Autodesk Fusion 360 part; units mm, degrees
(part 2 of 2)
extrude "Extrude1" add sketch "Sketch1" against normal blind 0.5 contours L0 L1 L2 L3 L4 L5 L6 L7 L8 L315 L316 | L18 L19 L20 L21 L38 L39 L40 L41 L42 L43 L44 L45 L46 L47 L48 L49 L50 L51 L52 L53 L54 L55 L56 L57 L58 L59 L60 L61 L62 L63 L64 L65 L66 L67 L68 L69 L70 L71 L72 L73 L74 L75 L76 L77 L78 L79 L80 L81 L82 L83 L84 L85 L86 L87 L88 L89 L90 L190 L191 L192 L193 L194 L195 L196 L197 L198 L199 L200 L201 L202 L203 L204 L205 L206 L207 L208 L209 L210 L211 L271 L272 L273 L274 L275 L276 L277 L278 L279 L280 L281 L282 L295 L296 L297 L298 L299 L300 L301 L313 L314 L315 L316 L329 L330 L331 L332 L333 L334 L335 L336 L337 L338 L339 L340 L341 L342 L343 L344 L345 L346 L347 L348 L349 L350 L351 L352 L353 L354 L355 L356 L357 L358 L359 L360 L361 L362 L363 L364 L411 L412 L413 L414 L415 L416 L417 L418 L419 L420 L421 L422 L423 L424 L425 L426 L427 L428 L429 L430 L431 L473 L474 L475 L476 L477 L478 L479 L480 L481 L482 L483 L484 L485 L486 L487 L488 L489 L490 L491 L492 L493 L494 L495 L496 L497 L498 L499 L500 L572 L573 L574 L575 L576 L577 L578 L579 L580 L581 L582 L583 L596 L597 L598 L599 L600 L601 L602 L603 L604 L605 L606 L607 L608 L609 L610 L611 L612 L613 L614 L615 L616 L617 L619 | L10 L11 L12 L316 | L313 L316 L317 L318 L319 L320 L321 L322 L323 L324 L325 L326 | L314 L620 L621 L622 L623 L624 L625 L626 L627 L628 L629 L630 L631 L632 | L313 L453 L454 L455 | L313 L314 L634 L635 L636 L637 L638 L639 | L313 L557 L558 L559 L560 L561 L562 L563 L564 L565 L566 L567 L568 L569 L570 L571 | L169 L170 L171 L172 L173 L174 L175 L176 L177 L178 L179 L180 L181 L182 L183 L184 L185 L186 L187 L188 L189 | L246 L247 L248 L249 L250 L251 L252 L253 | L263 L264 L265 L266 L267 L268 L269 L270 | L461 L462 L463 L464 L465 L466 L467 L468 L469 L470 L471 L472 | L692 L693 L694 L695 L696 L697 L702 L703 | L698 L699 L700 L701 makes body 1 at (43.6667, 42, 0) makes body 2 at (43.6667, 30.6667, 0) makes body 3 at (24, 8.3333, 0) makes body 4 at (55.6667, 34.6667, 0) makes body 5 at (24.3333, 29, 0)
extrude "Extrude2" add sketch "Sketch1" along normal blind 1 separate body contours L1 L2 L3 L4 L5 L6 L7 L8 L9 L10 L11 L12 L13 L14 L18 L19 L20 L21 L315 L316 | L38 L39 L40 L41 L42 L43 L44 L45 L46 L47 L48 L49 L50 L51 L52 L53 L54 L55 L56 L57 L58 L59 L60 L61 L62 L63 L64 L65 L66 L67 L68 L69 L70 L71 L72 L73 L74 L75 L76 L77 L78 L79 L80 L81 L82 L83 L84 L85 L86 L87 L88 L89 L90 L315 | L191 L192 L193 L194 L195 L196 L197 L198 L199 L200 L201 L202 L203 L204 L205 L206 L207 L208 L209 L210 L211 L315 | L313 L316 L319 L320 L321 L322 L323 L324 L325 L326 L327 L328 L329 L330 L331 L332 L333 L334 L335 L336 L337 L338 L339 L340 L341 L342 L343 L344 L345 L346 L347 L348 L349 L350 L351 L352 L353 L354 L355 L356 L357 L358 L359 L360 L361 L362 L363 L364 | L272 L273 L274 L275 L276 L277 L278 L279 L280 L281 L282 L315 | L295 L296 L297 L298 L299 L300 L301 L302 L303 L314 L315 | L313 L314 L597 L598 L599 L600 L601 L602 L603 L604 L605 L606 L607 L608 L609 L610 L611 L612 L613 L614 L615 L616 L617 L618 L619 L620 L621 L622 L623 L624 L625 L626 L627 L628 L629 L630 L631 L632 L633 L634 L635 L636 L637 L638 L639 | L313 L413 L414 L415 L416 L417 L418 L419 L420 L421 L422 L423 L424 L425 L426 L427 L428 L429 L430 L431 L453 L454 L455 | L313 L474 L475 L476 L477 L478 L479 L480 L481 L482 L483 L484 L485 L486 L487 L488 L489 L490 L491 L492 L493 L494 L495 L496 L497 L498 L499 L500 L557 L558 L559 L560 L561 L562 L563 L564 L565 L566 L567 L568 L569 L570 L571 | L313 L573 L574 L575 L576 L577 L578 L579 L580 L581 L582 L583 | L147 L148 L149 L150 L151 L152 L153 L154 L155 L156 L157 L158 L159 L160 L161 L162 L163 L164 L165 L166 L167 L168 | L238 L239 L240 L241 L242 L243 L244 L245 | L254 L255 L256 L257 L258 L259 L260 L261 L262 makes body 6 at (32.3333, 5, 0) makes body 7 at (63.3333, 32.3333, 0) makes body 8 at (21.3333, 30, 0) makes body 9 at (22, 36, 0) makes body 10 at (39.3333, 31, 0) makes body 11 at (54.3333, 6.3333, 0) makes body 12 at (18.3333, 5, 0) makes body 13 at (74.3333, 29.3333, 0) makes body 14 at (42.3333, 31, 0) makes body 15 at (1, 43, 0) makes body 16 at (42.3333, 40.6667, 0) makes body 17 at (76, 0.3333, 0) makes body 18 at (0.3333, 7.6667, 0)
extrude "Extrude3" cut sketch "Sketch1" against normal blind 1 contours L461 L462 L463 L464 L465 L466 L467 L468 L469 L470 L471 L472 bodies 3
extrude "Extrude4" add sketch "Sketch1" along normal blind 1 separate body contours L461 L462 L463 L464 L465 L466 L467 L468 L469 L470 L471 L472 makes body 19
extrude "Extrude5" add sketch "Sketch1" against normal blind 1 separate body contours L15 L16 L17 L22 L23 L24 L25 L26 L27 L28 L29 L30 L31 L32 L33 L34 L35 L36 L37 | L91 L92 L93 L94 L95 L96 L97 L98 L99 L100 L101 L102 L103 L104 L105 L106 L107 L108 L109 L110 L111 L112 L113 L114 L115 L116 L117 L118 L119 L120 L121 L122 L123 L124 L125 L126 L127 L128 L129 L130 L131 L132 L133 L134 L135 L136 L137 L138 L139 L140 L141 L142 L143 L144 L145 L146 | L212 L213 L214 L215 L216 L217 L218 L219 L220 L221 L222 L223 L224 L225 L226 L227 L228 L229 L230 L231 L232 L233 L234 L235 L236 L237 | L283 L284 L285 L286 L287 L288 L289 L290 L291 L292 L293 L294 | L304 L305 L306 L307 L308 L309 L310 L311 L312 | L365 L366 L367 L368 L369 L370 L371 L372 L373 L374 L375 L376 L377 L378 L379 L380 L381 L382 L383 L384 L385 L386 L387 L388 L389 L390 L391 L392 L393 L394 L395 L396 L397 L398 L399 L400 L401 L402 L403 L404 L405 L406 L407 L408 L409 L410 | L432 L433 L434 L435 L436 L437 L438 L439 L440 L441 L442 L443 L444 L445 L446 L447 L448 L449 L450 L451 L452 L456 L457 L458 L459 L460 | L501 L502 L503 L504 L505 L506 L507 L508 L509 L510 L511 L512 L513 L514 L515 L516 L517 L518 L519 L520 L521 L522 L523 L524 L525 L526 L527 L528 L529 L530 L531 L532 L533 L534 L535 L536 L537 L538 L539 L540 L541 L542 L543 L544 L545 L546 L547 L548 L549 L550 L551 L552 L553 L554 L555 L556 | L584 L585 L586 L587 L588 L589 L590 L591 L592 L593 L594 L595 | L640 L641 L642 L643 L644 L645 L646 L647 L648 L649 L650 L651 L652 L653 L654 L655 L656 L657 L658 L659 L660 L661 L662 L663 L664 L665 L666 L667 L668 L669 L670 L671 L672 L673 L674 L675 L676 L677 L678 L679 L680 L681 L682 L683 L684 L685 L686 L687 L688 L689 L690 L691 makes body 20 at (76, 46, 0) makes body 21 at (19, 35.3333, 0) makes body 22 at (19.6667, 6.6667, 0) makes body 23 at (9, 38.6667, 0) makes body 24 at (55.6667, 8.6667, 0) makes body 25 at (60.3333, 38, 0) makes body 26 at (34, 5, 0) makes body 27 at (11, 9.3333, 0) makes body 28 at (43, 24, 0) makes body 29 at (73, 2, 0)
extrude "Extrude6" add 14 faces at (1, 43, 0) (22, 36, 0) (21.3333, 30, 0) (39.3333, 31, 0) (42.3333, 31, 0) (42.3333, 40.6667, 0) (63.3333, 32.3333, 0) (74.3333, 29.3333, 0) (76, 0.3333, 0) (54.3333, 6.3333, 0) (32.3333, 5, 0) (21.3333, 10.3333, 0) (18.3333, 5, 0) (0.3333, 7.6667, 0) along direction (0, 0, -1) blind 0.5 on bodies 6 7 8 9 10 11 12 13 14 15 16 17 18 19 bodies 15 1 2 3 4 5 6 7 8 9 10 11 12 13 14 16 17 18 19 20 21 22 23 24 25 26 27 28 29
extrude "Extrude7" cut 10 faces at (11, 9.3333, -1) (19.6667, 6.6667, -1) (34, 5, -1) (55.6667, 8.6667, -1) (73, 2, -1) (60.3333, 38, -1) (76, 46, -1) (43, 24, -1) (19, 35.3333, -1) (9, 38.6667, -1) along direction (0, 0, 1) blind 0.5 on bodies 15 bodies 15
sketch "Sketch2" plane through (0, 0, 0) normal (0, 0, 1) x (1, 0, 0)
  line L0 (1, 14) -> (1, 15)
  line L1 (1, 15) -> (2, 15)
  line L2 (2, 15) -> (2, 16)
  line L3 (2, 16) -> (3, 16)
  line L4 (3, 16) -> (3, 17)
  line L5 (3, 17) -> (4, 17)
  line L6 (4, 17) -> (4, 18)
  line L7 (4, 18) -> (11, 18)
  line L8 (11, 18) -> (11, 14)
  line L9 (11, 14) -> (6, 14)
  line L10 (6, 14) -> (6, 13)
  line L11 (6, 13) -> (5, 13)
  line L12 (5, 13) -> (5, 12)
  line L13 (5, 12) -> (4, 12)
  line L14 (4, 12) -> (4, 6)
  line L15 (4, 6) -> (5, 6)
  line L16 (5, 6) -> (5, 5)
  line L17 (5, 5) -> (6, 5)
  line L18 (6, 5) -> (6, 4)
  line L19 (6, 4) -> (9, 4)
  line L20 (9, 4) -> (9, 5)
  line L21 (9, 5) -> (10, 5)
  line L22 (10, 5) -> (10, 6)
  line L23 (10, 6) -> (11, 6)
  line L24 (11, 6) -> (11, 7)
  line L25 (11, 7) -> (7, 7)
  line L26 (7, 7) -> (7, 11)
  line L27 (7, 11) -> (14, 11)
  line L28 (14, 11) -> (14, 3)
  line L29 (14, 3) -> (13, 3)
  line L30 (13, 3) -> (13, 2)
  line L31 (13, 2) -> (12, 2)
  line L32 (12, 2) -> (12, 1)
  line L33 (12, 1) -> (11, 1)
  line L34 (11, 1) -> (11, 0)
  line L35 (11, 0) -> (4, 0)
  line L36 (4, 0) -> (4, 1)
  line L37 (4, 1) -> (3, 1)
  line L38 (3, 1) -> (3, 2)
  line L39 (3, 2) -> (2, 2)
  line L40 (2, 2) -> (2, 3)
  line L41 (2, 3) -> (1, 3)
  line L42 (1, 3) -> (1, 4)
  line L43 (1, 4) -> (0, 4)
  line L44 (0, 4) -> (0, 14)
  line L45 (0, 14) -> (1, 14)
  line L46 (54, 0) -> (54, 18)
  line L47 (54, 18) -> (65, 18)
  line L48 (65, 18) -> (65, 14)
  line L49 (65, 14) -> (58, 14)
  line L50 (58, 14) -> (58, 11)
  line L51 (58, 11) -> (61, 11)
  line L52 (61, 11) -> (61, 7)
  line L53 (61, 7) -> (58, 7)
  line L54 (58, 7) -> (58, 4)
  line L55 (58, 4) -> (65, 4)
  line L56 (65, 4) -> (65, 0)
  line L57 (65, 0) -> (54, 0)
  line L58 (70, 43) -> (70, 48)
  line L59 (70, 48) -> (83, 48)
  line L60 (83, 48) -> (83, 43)
  line L61 (83, 43) -> (79, 43)
  line L62 (79, 43) -> (79, 22)
  line L63 (79, 22) -> (74, 22)
  line L64 (74, 22) -> (74, 43)
  line L65 (74, 43) -> (70, 43)
  line L66 (17, 45) -> (18, 45)
  line L67 (18, 45) -> (18, 46)
  line L68 (18, 46) -> (19, 46)
  line L69 (19, 46) -> (19, 47)
  line L70 (19, 47) -> (20, 47)
  line L71 (20, 47) -> (20, 48)
  line L72 (20, 48) -> (30, 48)
  line L73 (30, 48) -> (30, 47)
  line L74 (30, 47) -> (31, 47)
  line L75 (31, 47) -> (31, 46)
  line L76 (31, 46) -> (32, 46)
  line L77 (32, 46) -> (32, 45)
  line L78 (32, 45) -> (33, 45)
  line L79 (33, 45) -> (33, 40)
  line L80 (33, 40) -> (28, 40)
  line L81 (28, 40) -> (28, 42)
  line L82 (28, 42) -> (27, 42)
  line L83 (27, 42) -> (27, 43)
  line L84 (27, 43) -> (24, 43)
  line L85 (24, 43) -> (24, 42)
  line L86 (24, 42) -> (23, 42)
  line L87 (23, 42) -> (23, 41)
  line L88 (23, 41) -> (22, 41)
  line L89 (22, 41) -> (22, 37)
  line L90 (22, 37) -> (23, 37)
  line L91 (23, 37) -> (23, 38)
  line L92 (23, 38) -> (29, 38)
  line L93 (29, 38) -> (29, 37)
  line L94 (29, 37) -> (30, 37)
  line L95 (30, 37) -> (30, 36)
  line L96 (30, 36) -> (31, 36)
  line L97 (31, 36) -> (31, 35)
  line L98 (31, 35) -> (32, 35)
  line L99 (32, 35) -> (32, 34)
  line L100 (32, 34) -> (33, 34)
  line L101 (33, 34) -> (33, 25)
  line L102 (33, 25) -> (32, 25)
  line L103 (32, 25) -> (32, 24)
  line L104 (32, 24) -> (31, 24)
  line L105 (31, 24) -> (31, 23)
  line L106 (31, 23) -> (30, 23)
  line L107 (30, 23) -> (30, 22)
  line L108 (30, 22) -> (21, 22)
  line L109 (21, 22) -> (21, 23)
  line L110 (21, 23) -> (20, 23)
  line L111 (20, 23) -> (20, 24)
  line L112 (20, 24) -> (19, 24)
  line L113 (19, 24) -> (19, 25)
  line L114 (19, 25) -> (18, 25)
  line L115 (18, 25) -> (18, 26)
  line L116 (18, 26) -> (17, 26)
  line L117 (17, 26) -> (17, 45)
  line L118 (54, 22) -> (54, 27)
  line L119 (54, 27) -> (58, 27)
  line L120 (58, 27) -> (58, 43)
  line L121 (58, 43) -> (54, 43)
  line L122 (54, 43) -> (54, 48)
  line L123 (54, 48) -> (68, 48)
  line L124 (68, 48) -> (68, 43)
  line L125 (68, 43) -> (64, 43)
  line L126 (64, 43) -> (64, 27)
  line L127 (64, 27) -> (68, 27)
  line L128 (68, 27) -> (68, 22)
  line L129 (68, 22) -> (54, 22)
  line L130 (83, 18) -> (83, 14)
  line L131 (83, 14) -> (74, 14)
  line L132 (74, 14) -> (74, 12)
  line L133 (74, 12) -> (75, 12)
  line L134 (75, 12) -> (75, 11)
  line L135 (75, 11) -> (79, 11)
  line L136 (79, 11) -> (79, 10)
  line L137 (79, 10) -> (80, 10)
  line L138 (80, 10) -> (80, 9)
  line L139 (80, 9) -> (81, 9)
  line L140 (81, 9) -> (81, 8)
  line L141 (81, 8) -> (82, 8)
  line L142 (82, 8) -> (82, 7)
  line L143 (82, 7) -> (83, 7)
  line L144 (83, 7) -> (83, 3)
  line L145 (83, 3) -> (82, 3)
  line L146 (82, 3) -> (82, 2)
  line L147 (82, 2) -> (81, 2)
  line L148 (81, 2) -> (81, 1)
  line L149 (81, 1) -> (80, 1)
  line L150 (80, 1) -> (80, 0)
  line L151 (80, 0) -> (69, 0)
  line L152 (69, 0) -> (69, 4)
  line L153 (69, 4) -> (78, 4)
  line L154 (78, 4) -> (78, 6)
  line L155 (78, 6) -> (77, 6)
  line L156 (77, 6) -> (77, 7)
  line L157 (77, 7) -> (73, 7)
  line L158 (73, 7) -> (73, 8)
  line L159 (73, 8) -> (72, 8)
  line L160 (72, 8) -> (72, 9)
  line L161 (72, 9) -> (71, 9)
  line L162 (71, 9) -> (71, 10)
  line L163 (71, 10) -> (70, 10)
  line L164 (70, 10) -> (70, 11)
  line L165 (70, 11) -> (69, 11)
  line L166 (69, 11) -> (69, 15)
  line L167 (69, 15) -> (70, 15)
  line L168 (70, 15) -> (70, 16)
  line L169 (70, 16) -> (71, 16)
  line L170 (71, 16) -> (71, 17)
  line L171 (71, 17) -> (72, 17)
  line L172 (72, 17) -> (72, 18)
  line L173 (72, 18) -> (83, 18)
  line L174 (47, 0) -> (47, 12)
  line L175 (47, 12) -> (46, 12)
  line L176 (46, 12) -> (46, 13)
  line L177 (46, 13) -> (44, 13)
  line L178 (44, 13) -> (44, 12)
  line L179 (44, 12) -> (43, 12)
  line L180 (43, 12) -> (43, 7)
  line L181 (43, 7) -> (40, 7)
  line L182 (40, 7) -> (40, 12)
  line L183 (40, 12) -> (39, 12)
  line L184 (39, 12) -> (39, 13)
  line L185 (39, 13) -> (37, 13)
  line L186 (37, 13) -> (37, 12)
  line L187 (37, 12) -> (36, 12)
  line L188 (36, 12) -> (36, 0)
  line L189 (36, 0) -> (32, 0)
  line L190 (32, 0) -> (32, 14)
  line L191 (32, 14) -> (33, 14)
  line L192 (33, 14) -> (33, 15)
  line L193 (33, 15) -> (34, 15)
  line L194 (34, 15) -> (34, 16)
  line L195 (34, 16) -> (35, 16)
  line L196 (35, 16) -> (35, 17)
  line L197 (35, 17) -> (36, 17)
  line L198 (36, 17) -> (36, 18)
  line L199 (36, 18) -> (40, 18)
  line L200 (40, 18) -> (40, 17)
  line L201 (40, 17) -> (41, 17)
  line L202 (41, 17) -> (41, 16)
  line L203 (41, 16) -> (42, 16)
  line L204 (42, 16) -> (42, 17)
  line L205 (42, 17) -> (43, 17)
  line L206 (43, 17) -> (43, 18)
  line L207 (43, 18) -> (47, 18)
  line L208 (47, 18) -> (47, 17)
  line L209 (47, 17) -> (48, 17)
  line L210 (48, 17) -> (48, 16)
  line L211 (48, 16) -> (49, 16)
  line L212 (49, 16) -> (49, 15)
  line L213 (49, 15) -> (50, 15)
  line L214 (50, 15) -> (50, 14)
  line L215 (50, 14) -> (51, 14)
  line L216 (51, 14) -> (51, 0)
  line L217 (51, 0) -> (47, 0)
  line L218 (18, 0) -> (18, 14)
  line L219 (18, 14) -> (19, 14)
  line L220 (19, 14) -> (19, 15)
  line L221 (19, 15) -> (20, 15)
  line L222 (20, 15) -> (20, 16)
  line L223 (20, 16) -> (21, 16)
  line L224 (21, 16) -> (21, 17)
  line L225 (21, 17) -> (22, 17)
  line L226 (22, 17) -> (22, 18)
  line L227 (22, 18) -> (25, 18)
  line L228 (25, 18) -> (25, 17)
  line L229 (25, 17) -> (26, 17)
  line L230 (26, 17) -> (26, 16)
  line L231 (26, 16) -> (27, 16)
  line L232 (27, 16) -> (27, 15)
  line L233 (27, 15) -> (28, 15)
  line L234 (28, 15) -> (28, 14)
  line L235 (28, 14) -> (29, 14)
  line L236 (29, 14) -> (29, 0)
  line L237 (29, 0) -> (25, 0)
  line L238 (25, 0) -> (25, 4)
  line L239 (25, 4) -> (22, 4)
  line L240 (22, 4) -> (22, 0)
  line L241 (22, 0) -> (18, 0)
  line L242 (0, 44) -> (1, 44)
  line L243 (1, 44) -> (1, 45)
  line L244 (1, 45) -> (2, 45)
  line L245 (2, 45) -> (2, 46)
  line L246 (2, 46) -> (3, 46)
  line L247 (3, 46) -> (3, 47)
  line L248 (3, 47) -> (4, 47)
  line L249 (4, 47) -> (4, 48)
  line L250 (4, 48) -> (11, 48)
  line L251 (11, 48) -> (11, 27)
  line L252 (11, 27) -> (15, 27)
  line L253 (15, 27) -> (15, 22)
  line L254 (15, 22) -> (0, 22)
  line L255 (0, 22) -> (0, 27)
  line L256 (0, 27) -> (6, 27)
  line L257 (6, 27) -> (6, 42)
  line L258 (6, 42) -> (0, 42)
  line L259 (0, 42) -> (0, 44)
  line L260 (-1, 49) -> (-1, -1)
  line L261 (-1, -1) -> (84, -1)
  line L262 (84, -1) -> (84, 49)
  line L263 (84, 49) -> (-1, 49)
  line L264 (49, 47) -> (50, 47)
  line L265 (50, 47) -> (50, 46)
  line L266 (50, 46) -> (51, 46)
  line L267 (51, 46) -> (51, 37)
  line L268 (51, 37) -> (50, 37)
  line L269 (50, 37) -> (50, 36)
  line L270 (50, 36) -> (49, 36)
  line L271 (49, 36) -> (49, 35)
  line L272 (49, 35) -> (50, 35)
  line L273 (50, 35) -> (50, 34)
  line L274 (50, 34) -> (51, 34)
  line L275 (51, 34) -> (51, 25)
  line L276 (51, 25) -> (50, 25)
  line L277 (50, 25) -> (50, 24)
  line L278 (50, 24) -> (49, 24)
  line L279 (49, 24) -> (49, 23)
  line L280 (49, 23) -> (48, 23)
  line L281 (48, 23) -> (48, 22)
  line L282 (48, 22) -> (39, 22)
  line L283 (39, 22) -> (39, 48)
  line L284 (39, 48) -> (49, 48)
  line L285 (49, 48) -> (49, 47)
  line L286 (-2, -2) -> (85, -2)
  line L287 (85, -2) -> (85, 50)
  line L288 (85, 50) -> (-2, 50)
  line L289 (-2, 50) -> (-2, -2)
  constraint horizontal L286
  constraint vertical L287
  constraint horizontal L288
  constraint vertical L289
extrude "Extrude8" add sketch "Sketch2" against normal blind 0.5 contours L286 L287 L288 L289 bodies 15
sketch "Sketch3" plane through (0, 0, 0) normal (0, 0, 1) x (1, 0, 0)
  line L0 (-2, 50) -> (-2, -2)
  line L1 (-2, -2) -> (85, -2)
  line L2 (85, -2) -> (85, 50)
  line L3 (85, 50) -> (-2, 50)
  line L4 (1, 14) -> (1, 15)
  line L5 (1, 15) -> (2, 15)
  line L6 (2, 15) -> (2, 16)
  line L7 (2, 16) -> (3, 16)
  line L8 (3, 16) -> (3, 17)
  line L9 (3, 17) -> (4, 17)
  line L10 (4, 17) -> (4, 18)
  line L11 (4, 18) -> (11, 18)
  line L12 (11, 18) -> (11, 14)
  line L13 (11, 14) -> (6, 14)
  line L14 (6, 14) -> (6, 13)
  line L15 (6, 13) -> (5, 13)
  line L16 (5, 13) -> (5, 12)
  line L17 (5, 12) -> (4, 12)
  line L18 (4, 12) -> (4, 6)
  line L19 (4, 6) -> (5, 6)
  line L20 (5, 6) -> (5, 5)
  line L21 (5, 5) -> (6, 5)
  line L22 (6, 5) -> (6, 4)
  line L23 (6, 4) -> (9, 4)
  line L24 (9, 4) -> (9, 5)
  line L25 (9, 5) -> (10, 5)
  line L26 (10, 5) -> (10, 6)
  line L27 (10, 6) -> (11, 6)
  line L28 (11, 6) -> (11, 7)
  line L29 (11, 7) -> (7, 7)
  line L30 (7, 7) -> (7, 11)
  line L31 (7, 11) -> (14, 11)
  line L32 (14, 11) -> (14, 3)
  line L33 (14, 3) -> (13, 3)
  line L34 (13, 3) -> (13, 2)
  line L35 (13, 2) -> (12, 2)
  line L36 (12, 2) -> (12, 1)
  line L37 (12, 1) -> (11, 1)
  line L38 (11, 1) -> (11, 0)
  line L39 (11, 0) -> (4, 0)
  line L40 (4, 0) -> (4, 1)
  line L41 (4, 1) -> (3, 1)
  line L42 (3, 1) -> (3, 2)
  line L43 (3, 2) -> (2, 2)
  line L44 (2, 2) -> (2, 3)
  line L45 (2, 3) -> (1, 3)
  line L46 (1, 3) -> (1, 4)
  line L47 (1, 4) -> (0, 4)
  line L48 (0, 4) -> (0, 14)
  line L49 (0, 14) -> (1, 14)
  line L50 (54, 0) -> (54, 18)
  line L51 (54, 18) -> (65, 18)
  line L52 (65, 18) -> (65, 14)
  line L53 (65, 14) -> (58, 14)
  line L54 (58, 14) -> (58, 11)
  line L55 (58, 11) -> (61, 11)
  line L56 (61, 11) -> (61, 7)
  line L57 (61, 7) -> (58, 7)
  line L58 (58, 7) -> (58, 4)
  line L59 (58, 4) -> (65, 4)
  line L60 (65, 4) -> (65, 0)
  line L61 (65, 0) -> (54, 0)
  line L62 (70, 43) -> (70, 48)
  line L63 (70, 48) -> (83, 48)
  line L64 (83, 48) -> (83, 43)
  line L65 (83, 43) -> (79, 43)
  line L66 (79, 43) -> (79, 22)
  line L67 (79, 22) -> (74, 22)
  line L68 (74, 22) -> (74, 43)
  line L69 (74, 43) -> (70, 43)
  line L70 (17, 45) -> (18, 45)
  line L71 (18, 45) -> (18, 46)
  line L72 (18, 46) -> (19, 46)
  line L73 (19, 46) -> (19, 47)
  line L74 (19, 47) -> (20, 47)
  line L75 (20, 47) -> (20, 48)
  line L76 (20, 48) -> (30, 48)
  line L77 (30, 48) -> (30, 47)
  line L78 (30, 47) -> (31, 47)
  line L79 (31, 47) -> (31, 46)
  line L80 (31, 46) -> (32, 46)
  line L81 (32, 46) -> (32, 45)
  line L82 (32, 45) -> (33, 45)
  line L83 (33, 45) -> (33, 40)
  line L84 (33, 40) -> (28, 40)
  line L85 (28, 40) -> (28, 42)
  line L86 (28, 42) -> (27, 42)
  line L87 (27, 42) -> (27, 43)
  line L88 (27, 43) -> (24, 43)
  line L89 (24, 43) -> (24, 42)
  line L90 (24, 42) -> (23, 42)
  line L91 (23, 42) -> (23, 41)
  line L92 (23, 41) -> (22, 41)
  line L93 (22, 41) -> (22, 37)
  line L94 (22, 37) -> (23, 37)
  line L95 (23, 37) -> (23, 38)
  line L96 (23, 38) -> (29, 38)
  line L97 (29, 38) -> (29, 37)
  line L98 (29, 37) -> (30, 37)
  line L99 (30, 37) -> (30, 36)
  line L100 (30, 36) -> (31, 36)
  line L101 (31, 36) -> (31, 35)
  line L102 (31, 35) -> (32, 35)
  line L103 (32, 35) -> (32, 34)
  line L104 (32, 34) -> (33, 34)
  line L105 (33, 34) -> (33, 25)
  line L106 (33, 25) -> (32, 25)
  line L107 (32, 25) -> (32, 24)
  line L108 (32, 24) -> (31, 24)
  line L109 (31, 24) -> (31, 23)
  line L110 (31, 23) -> (30, 23)
  line L111 (30, 23) -> (30, 22)
  line L112 (30, 22) -> (21, 22)
  line L113 (21, 22) -> (21, 23)
  line L114 (21, 23) -> (20, 23)
  line L115 (20, 23) -> (20, 24)
  line L116 (20, 24) -> (19, 24)
  line L117 (19, 24) -> (19, 25)
  line L118 (19, 25) -> (18, 25)
  line L119 (18, 25) -> (18, 26)
  line L120 (18, 26) -> (17, 26)
  line L121 (17, 26) -> (17, 45)
  line L122 (54, 22) -> (54, 27)
  line L123 (54, 27) -> (58, 27)
  line L124 (58, 27) -> (58, 43)
  line L125 (58, 43) -> (54, 43)
  line L126 (54, 43) -> (54, 48)
  line L127 (54, 48) -> (68, 48)
  line L128 (68, 48) -> (68, 43)
  line L129 (68, 43) -> (64, 43)
  line L130 (64, 43) -> (64, 27)
  line L131 (64, 27) -> (68, 27)
  line L132 (68, 27) -> (68, 22)
  line L133 (68, 22) -> (54, 22)
  line L134 (83, 18) -> (83, 14)
  line L135 (83, 14) -> (74, 14)
  line L136 (74, 14) -> (74, 12)
  line L137 (74, 12) -> (75, 12)
  line L138 (75, 12) -> (75, 11)
  line L139 (75, 11) -> (79, 11)
  line L140 (79, 11) -> (79, 10)
  line L141 (79, 10) -> (80, 10)
  line L142 (80, 10) -> (80, 9)
  line L143 (80, 9) -> (81, 9)
  line L144 (81, 9) -> (81, 8)
  line L145 (81, 8) -> (82, 8)
  line L146 (82, 8) -> (82, 7)
  line L147 (82, 7) -> (83, 7)
  line L148 (83, 7) -> (83, 3)
  line L149 (83, 3) -> (82, 3)
  line L150 (82, 3) -> (82, 2)
  line L151 (82, 2) -> (81, 2)
  line L152 (81, 2) -> (81, 1)
  line L153 (81, 1) -> (80, 1)
  line L154 (80, 1) -> (80, 0)
  line L155 (80, 0) -> (69, 0)
  line L156 (69, 0) -> (69, 4)
  line L157 (69, 4) -> (78, 4)
  line L158 (78, 4) -> (78, 6)
  line L159 (78, 6) -> (77, 6)
  line L160 (77, 6) -> (77, 7)
  line L161 (77, 7) -> (73, 7)
  line L162 (73, 7) -> (73, 8)
  line L163 (73, 8) -> (72, 8)
  line L164 (72, 8) -> (72, 9)
  line L165 (72, 9) -> (71, 9)
  line L166 (71, 9) -> (71, 10)
  line L167 (71, 10) -> (70, 10)
  line L168 (70, 10) -> (70, 11)
  line L169 (70, 11) -> (69, 11)
  line L170 (69, 11) -> (69, 15)
  line L171 (69, 15) -> (70, 15)
  line L172 (70, 15) -> (70, 16)
  line L173 (70, 16) -> (71, 16)
  line L174 (71, 16) -> (71, 17)
  line L175 (71, 17) -> (72, 17)
  line L176 (72, 17) -> (72, 18)
  line L177 (72, 18) -> (83, 18)
  line L178 (47, 0) -> (47, 12)
  line L179 (47, 12) -> (46, 12)
  line L180 (46, 12) -> (46, 13)
  line L181 (46, 13) -> (44, 13)
  line L182 (44, 13) -> (44, 12)
  line L183 (44, 12) -> (43, 12)
  line L184 (43, 12) -> (43, 7)
  line L185 (43, 7) -> (40, 7)
  line L186 (40, 7) -> (40, 12)
  line L187 (40, 12) -> (39, 12)
  line L188 (39, 12) -> (39, 13)
  line L189 (39, 13) -> (37, 13)
  line L190 (37, 13) -> (37, 12)
  line L191 (37, 12) -> (36, 12)
  line L192 (36, 12) -> (36, 0)
  line L193 (36, 0) -> (32, 0)
  line L194 (32, 0) -> (32, 14)
  line L195 (32, 14) -> (33, 14)
  line L196 (33, 14) -> (33, 15)
  line L197 (33, 15) -> (34, 15)
  line L198 (34, 15) -> (34, 16)
  line L199 (34, 16) -> (35, 16)
  line L200 (35, 16) -> (35, 17)
  line L201 (35, 17) -> (36, 17)
  line L202 (36, 17) -> (36, 18)
  line L203 (36, 18) -> (40, 18)
  line L204 (40, 18) -> (40, 17)
  line L205 (40, 17) -> (41, 17)
  line L206 (41, 17) -> (41, 16)
  line L207 (41, 16) -> (42, 16)
  line L208 (42, 16) -> (42, 17)
  line L209 (42, 17) -> (43, 17)
  line L210 (43, 17) -> (43, 18)
  line L211 (43, 18) -> (47, 18)
  line L212 (47, 18) -> (47, 17)
  line L213 (47, 17) -> (48, 17)
  line L214 (48, 17) -> (48, 16)
  line L215 (48, 16) -> (49, 16)
  line L216 (49, 16) -> (49, 15)
  line L217 (49, 15) -> (50, 15)
  line L218 (50, 15) -> (50, 14)
  line L219 (50, 14) -> (51, 14)
  line L220 (51, 14) -> (51, 0)
  line L221 (51, 0) -> (47, 0)
  line L222 (18, 0) -> (18, 14)
  line L223 (18, 14) -> (19, 14)
  line L224 (19, 14) -> (19, 15)
  line L225 (19, 15) -> (20, 15)
  line L226 (20, 15) -> (20, 16)
  line L227 (20, 16) -> (21, 16)
  line L228 (21, 16) -> (21, 17)
  line L229 (21, 17) -> (22, 17)
  line L230 (22, 17) -> (22, 18)
  line L231 (22, 18) -> (25, 18)
  line L232 (25, 18) -> (25, 17)
  line L233 (25, 17) -> (26, 17)
  line L234 (26, 17) -> (26, 16)
  line L235 (26, 16) -> (27, 16)
  line L236 (27, 16) -> (27, 15)
  line L237 (27, 15) -> (28, 15)
  line L238 (28, 15) -> (28, 14)
  line L239 (28, 14) -> (29, 14)
  line L240 (29, 14) -> (29, 0)
  line L241 (29, 0) -> (25, 0)
  line L242 (25, 0) -> (25, 4)
  line L243 (25, 4) -> (22, 4)
  line L244 (22, 4) -> (22, 0)
  line L245 (22, 0) -> (18, 0)
  line L246 (0, 44) -> (1, 44)
  line L247 (1, 44) -> (1, 45)
  line L248 (1, 45) -> (2, 45)
  line L249 (2, 45) -> (2, 46)
  line L250 (2, 46) -> (3, 46)
  line L251 (3, 46) -> (3, 47)
  line L252 (3, 47) -> (4, 47)
  line L253 (4, 47) -> (4, 48)
  line L254 (4, 48) -> (11, 48)
  line L255 (11, 48) -> (11, 27)
  line L256 (11, 27) -> (15, 27)
  line L257 (15, 27) -> (15, 22)
  line L258 (15, 22) -> (0, 22)
  line L259 (0, 22) -> (0, 27)
  line L260 (0, 27) -> (6, 27)
  line L261 (6, 27) -> (6, 42)
  line L262 (6, 42) -> (0, 42)
  line L263 (0, 42) -> (0, 44)
  line L264 (49, 47) -> (50, 47)
  line L265 (50, 47) -> (50, 46)
  line L266 (50, 46) -> (51, 46)
  line L267 (51, 46) -> (51, 37)
  line L268 (51, 37) -> (50, 37)
  line L269 (50, 37) -> (50, 36)
  line L270 (50, 36) -> (49, 36)
  line L271 (49, 36) -> (49, 35)
  line L272 (49, 35) -> (50, 35)
  line L273 (50, 35) -> (50, 34)
  line L274 (50, 34) -> (51, 34)
  line L275 (51, 34) -> (51, 25)
  line L276 (51, 25) -> (50, 25)
  line L277 (50, 25) -> (50, 24)
  line L278 (50, 24) -> (49, 24)
  line L279 (49, 24) -> (49, 23)
  line L280 (49, 23) -> (48, 23)
  line L281 (48, 23) -> (48, 22)
  line L282 (48, 22) -> (39, 22)
  line L283 (39, 22) -> (39, 48)
  line L284 (39, 48) -> (49, 48)
  line L285 (49, 48) -> (49, 47)
  line L286 (-2, 50) -> (3, 50)
  line L287 (3, 50) -> (3, 46)
  line L288 (3, 46) -> (-2, 46)
  line L289 (-2, 46) -> (-2, 50)
  circle A0 centre (0.5, 48) radius 1.5
  dimension "d41" = 3
  constraint horizontal L286
  constraint vertical L287
  constraint horizontal L288
  constraint vertical L289
  constraint coincident L250.end L251.start
  constraint coincident L0.start L3.end
  measures "d41" diameter of A0
extrude "Extrude9" cut sketch "Sketch3" against normal blind 0.5 contours A0 bodies 15
